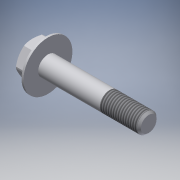
# Autodesk Inventor part: Bolt
Saved by Autodesk Inventor 2019 (Build 230136000, 136)
## iProperties
Created: 2010-08-06
Part Number: Bolt
Document SubType Name: Modeling
Designer: nguyenducthang
Density: 1 g/cm^3
Mass: 0.0491976 g
Surface Area: 1.21375 cm^2
Volume: 0.0491976 cm^3
Material: Generic
Appearance: Cool White
Author: nguyenducthang
Autodesk Inventor part; units mm, degrees
ref_plane "YZ Plane" through (0, 0, 0) normal (1, 0, 0) x (0, 1, 0)
ref_plane "XZ Plane" through (0, 0, 0) normal (0, 1, 0) x (-1, 0, 0)
ref_plane "XY Plane" through (0, 0, 0) normal (0, 0, 1) x (1, 0, 0)
sketch "Sketch15" plane through (0, 0, 0) normal (0, 0, 1) x (1, 0, 0)
  line L0 (0, 0) -> (0, 1.4)
  line L1 (0.2309, 1.8) -> (1.5, 1.8)
  line L2 (1.5, 1.8) -> (1.5, 2.5)
  line L3 (1.5, 2.5) -> (1.7, 2.5)
  line L4 (1.7, 2.5) -> (1.7, 1)
  line L5 (1.7, 1) -> (12, 1)
  line L6 (12, 0) -> (0, 0)
  line L7 (0.2309, 1.8) -> (0, 1.4)
  line L8 (12, 1) -> (12, 0)
  dimension "d78" = 0.2
  dimension "d83" = 30
  dimension "d84" = 1
  dimension "d86" = 0.4
  dimension "d87" = 1.8
  dimension "d89" = 1.5
  dimension "d90" = 2.5
  dimension "d115" = 12
  constraints: 18 end point, 5 parallel, 1 perpendicular, 1 vertical, 1 other
  measures "d78" distance of L2.end L3.end
  measures "d83" angle of L0 L7
  measures "d84" distance between parallel lines of L5 L6
  measures "d86" distance from line of L0.end L1
  measures "d87" distance between parallel lines of L1 L6
  measures "d89" distance between parallel lines of L2 L0
  measures "d90" distance between parallel lines of L3 L6
  measures "d115" distance of L6.start L0.start
revolve "Revolution1" add sketch "Sketch15" angle 360 about axis through (12, 0, 0) along (-1, 0, 0)
thread "Thread2" size "M2x0.25" class "6g" standard "ANSI Metric M Profile" length 4
sketch "Sketch16" plane through (0, 0, 0) normal (-1, 0, 0) x (0, 0, 1)
  circle A0 centre (0, 0) radius 1.4 projected
  line L0 (0.9238, 1.6) -> (1.8475, 0)
  line L1 (1.8475, 0) -> (0.9238, -1.6)
  line L2 (0.9238, -1.6) -> (-0.9238, -1.6)
  line L3 (-0.9238, -1.6) -> (-1.8475, 0)
  line L4 (-1.8475, 0) -> (-0.9238, 1.6)
  line L5 (-0.9238, 1.6) -> (0.9238, 1.6)
  circle A1 centre (0, 0) radius 2.6573
  dimension "d104" = 3.2
  constraints: 12 end point, 2 coincident, 1 centre point, 13 other
  measures "d104" distance between parallel lines of L5 L2
extrude "Extrusion15" cut sketch "Sketch16" against normal up to surface (1.5 mm away) contours A1
chamfer "Chamfer5" distance 0.2 angle 45 1 edges at (12, -1, 0)
body "Solid1"
